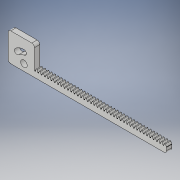
# Autodesk Inventor part: CameraBaseLeft
Saved by Autodesk Inventor 2019 (Build 230136000, 136)
## iProperties
Created: 2019-07-15
Part Number: CameraBaseLeft
Material: Generic
Document SubType Name: Modeling
Designer: aorfi
Density: 1 g/cm^3
Appearance: Default
Author: aorfi
Autodesk Inventor part; units mm, degrees
ref_plane "YZ Plane" through (0, 0, 0) normal (1, 0, 0) x (0, 1, 0)
ref_plane "XZ Plane" through (0, 0, 0) normal (0, 1, 0) x (-1, 0, 0)
ref_plane "XY Plane" through (0, 0, 0) normal (0, 0, 1) x (1, 0, 0)
sketch "Sketch1" plane through (0, 0, 0) normal (0, 0, 1) x (1, 0, 0)
  line L0 (-60, -10.7625) -> (60, -10.7625)
  line L1 (60, -10.7625) -> (60, 10.7625)
  line L2 (60, 10.7625) -> (-60, 10.7625)
  line L3 (-60, 10.7625) -> (-60, -10.7625)
  line L4 (-60, -10.7625) -> (60, 10.7625) construction
  line L5 (60, -10.7625) -> (-60, 10.7625) construction
  point P0 (0, 0)
  dimension "d3" = 21.525
  dimension "d26" = 120
  constraints: 12 end point, 2 midpoint, 2 parallel, 1 horizontal, 1 perpendicular
  measures "d3" distance of L2.end L0.start
  measures "d26" distance of L0.start L0.end
extrude "Extrusion1" add sketch "Sketch1" along normal mid plane 4
sketch "Sketch2" plane through (0, 0, -2) normal (0, 0, -1) x (-1, 0, 0)
  circle A0 centre (48, -5.7625) radius 2.5
  arc A1 (48, 3.6361) -> (48, -0.1612) centre (48, 1.7375) ccw
  line L0 (48, 1.7375) -> (48, -5.7625) construction
  line L1 (48, -5.7625) -> (53.3033, -5.7625) construction
  circle A2 centre (48, -5.7625) radius 7.5 construction
  arc A3 (51.9608, -1.8017) -> (54.6458, 0.8833) centre (53.3033, -0.4592) ccw
  arc A4 (54.6458, 0.8833) -> (48, 3.6361) centre (48, -5.7625) ccw
  arc A5 (51.9608, -1.8017) -> (48, -0.1612) centre (48, -5.7625) ccw
  line L2 (60, -10.7625) -> (60, 10.7625) construction
  line L3 (0, -15) -> (0, 15) construction
  line L4 (60, 10.7625) -> (-60, 10.7625) projected
  line L5 (-60, -10.7625) -> (60, -10.7625) projected
  line L6 (48, -5.7625) -> (53.3033, -0.4592) construction
  line L7 (53.3033, -0.4592) -> (53.3033, -5.7625) construction
  point P0 (0, 0)
  point P1 (60, 0)
  dimension "d4" = 5
  dimension "d5" = 3.7973
  dimension "d7" = 3.7973
  dimension "d8" = 15
  dimension "d9" = 12
  dimension "d57" = 5
  constraints: 10 end point, 10 point on circle, 6 centre point, 4 coincident, 2 tangent, 2 vertical, 1 horizontal, 1 midpoint, 1 perpendicular, 1 point on line, 1 vertical alignment
  measures "d4" diameter of A0
  measures "d5" diameter of A1
  measures "d7" diameter of A3
  measures "d8" diameter of A2
  measures "d9" distance from line of L0.end L2
  measures "d57" distance from line of L5 L0.end
extrude "Extrusion2" cut sketch "Sketch2" against normal through all
sketch "Sketch6" plane through (0, 0, 2) normal (0, 0, -1) x (-1, 0, 0)
  line L0 (60, 10.7625) -> (-60, 10.7625) projected
  line L1 (60, -10.7625) -> (-60, -10.7625) projected
  arc A0 (36.8815, -6.3788) -> (37.0623, -6.5596) centre (37.0623, -6.3788) ccw
  line L2 (37.0623, -6.5596) -> (37.3256, -6.5596)
  arc A1 (37.3256, -6.5596) -> (37.4955, -6.4406) centre (37.3256, -6.3788) ccw
  line L3 (37.4955, -6.4406) -> (38.1062, -4.7625)
  line L4 (38.7753, -4.7625) -> (38.1062, -4.7625)
  line L5 (38.7753, -4.7625) -> (39.386, -6.4406)
  arc A2 (39.386, -6.4406) -> (39.5559, -6.5596) centre (39.5559, -6.3788) ccw
  line L6 (39.5559, -6.5596) -> (39.8192, -6.5596)
  line L7 (39.5559, -6.3788) -> (37.3256, -6.3788) construction
  line L8 (36.8815, -6.3788) -> (36.8815, 10.7625)
  line L9 (36.8815, 10.7625) -> (40, 10.7625)
  line L10 (40, 10.7625) -> (40, -6.3788)
  arc A3 (39.8192, -6.5596) -> (40, -6.3788) centre (39.8192, -6.3788) ccw
  line L11 (60, 10.7625) -> (60, -10.7625) projected
  line L12 (-60, 10.7625) -> (60, 10.7625) projected
  point P0 (0, 0)
  point P1 (38.4407, -4.7625)
  point P2 (38.4407, -6.3788)
  dimension "d58" = 0.1808
  dimension "d59" = 1.7971
  dimension "d60" = 0.2633
  dimension "d61" = 0.669
  dimension "d62" = 2.2303
  dimension "d64" = 20
  dimension "d66" = 6
  constraints: 18 end point, 8 point on circle, 8 tangent, 5 horizontal, 4 centre point, 3 equal radius, 2 collinear, 2 midpoint, 1 perpendicular, 1 vertical, 1 vertical alignment
  measures "d58" radius of A1
  measures "d59" distance between parallel lines of L2 L4
  measures "d60" distance of L2.start L2.end
  measures "d61" distance of L4.start L3.end
  measures "d62" distance of L7.start L7.end
  measures "d64" distance between parallel lines of L11 L10
  measures "d66" distance between parallel lines of L1 L4
extrude "Extrusion4" cut sketch "Sketch6" along normal through all
pattern_linear "Rectangular Pattern1" count 40 spacing 2.4936 along (1, 0, 0) of "Extrusion4"
fillet "Fillet1" radius 2 4 edges at (-60, 10.7625, 0) (-60, -10.7625, 0) (60, -10.7625, 0) (-40, 10.7625, 0)
equation "\"d7\" = d5"
body "Solid1"
